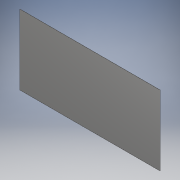
# Autodesk Inventor part: SteelTankSideandBottom
Saved by Autodesk Inventor 2019 (Build 230136000, 136)
## iProperties
Created: 2021-05-18
Part Number: SteelTankSideandBottom
Material: Generic
Document SubType Name: Modeling
Designer: jamieson-bl
Density: 1 g/cm^3
Appearance: Default
Author: jamieson-bl
Autodesk Inventor part; units mm, degrees
ref_plane "YZ Plane" through (0, 0, 0) normal (1, 0, 0) x (0, 1, 0)
ref_plane "XZ Plane" through (0, 0, 0) normal (0, 1, 0) x (-1, 0, 0)
ref_plane "XY Plane" through (0, 0, 0) normal (0, 0, 1) x (1, 0, 0)
sketch "Sketch1" plane through (0, 0, 0) normal (0, 0, 1) x (1, 0, 0)
  line L0 (1524, -762) -> (-1524, -762)
  line L1 (-1524, -762) -> (-1524, 762)
  line L2 (-1524, 762) -> (1524, 762)
  line L3 (1524, 762) -> (1524, -762)
  line L4 (1524, -762) -> (-1524, 762) construction
  line L5 (-1524, -762) -> (1524, 762) construction
  point P0 (0, 0)
  dimension "d0" = 3048
  dimension "d1" = 1524
  constraints: 12 end point, 2 midpoint, 2 parallel, 1 horizontal, 1 perpendicular
  measures "d0" distance of L1.end L2.end
  measures "d1" distance of L0.end L1.end
extrude "Extrusion1" add sketch "Sketch1" along normal blind 2.7432
